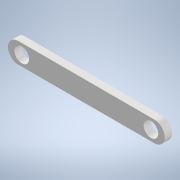
# Autodesk Inventor part: crank part
Saved by Autodesk Inventor 2022 (Build 260153070, 153G)
## iProperties
Created: 2021-07-24
Part Number: crank part
Material: Generic
Document SubType Name: Sheet Metal
Designer: DELL
Density: 1 g/cm^3
Sheet Metal Rule: Default
Appearance: Default
Author: DELL
Autodesk Inventor part; units mm, degrees
ref_plane "YZ Plane" through (0, 0, 0) normal (1, 0, 0) x (0, 1, 0)
ref_plane "XZ Plane" through (0, 0, 0) normal (0, 1, 0) x (-1, 0, 0)
ref_plane "XY Plane" through (0, 0, 0) normal (0, 0, 1) x (1, 0, 0)
sketch "Sketch1" plane through (0, 0, 0) normal (0, 0, 1) x (1, 0, 0)
  line L0 (-87.95, 8.89) -> (87.95, 8.89)
  line L1 (87.95, 8.89) -> (87.95, -8.89)
  line L2 (87.95, -8.89) -> (-87.95, -8.89)
  line L3 (-87.95, -8.89) -> (-87.95, 8.89)
  line L4 (-87.95, 8.89) -> (87.95, -8.89) construction
  line L5 (87.95, 8.89) -> (-87.95, -8.89) construction
  point P0 (0, 0)
  dimension "d0" = 175.9
  dimension "d1" = 17.78
  constraints: 12 end point, 2 midpoint, 2 parallel, 1 horizontal, 1 perpendicular
  measures "d0" distance of L1.end L2.end
  measures "d1" distance of L0.end L1.end
extrude "Extrusion1" add sketch "Sketch1" along normal blind 6.35
fillet "Fillet1" radius 8.89 1 edges at (87.95, 8.89, 3.175)
fillet "Fillet2" radius 8.89 1 edges at (87.95, -8.89, 3.175)
fillet "Fillet3" radius 8.89 1 edges at (-87.95, -8.89, 3.175)
fillet "Fillet4" radius 8.89 1 edges at (-87.95, 8.89, 3.175)
sketch "Sketch2" plane through (0, 0, 6.35) normal (0, 0, 1) x (1, 0, 0)
  arc A0 (79.06, -8.89) -> (79.06, 8.89) centre (79.06, 0) ccw projected
  circle A1 centre (-75.96, 0) radius 6.35
  circle A2 centre (75.96, 0) radius 6.35
  arc A3 (-79.06, 8.89) -> (-79.06, -8.89) centre (-79.06, 0) ccw projected
  point P0 (0, 0)
  dimension "d10" = 12.7
  dimension "d12" = 12.7
  dimension "d13" = 3.1
  dimension "d14" = 3.1
  constraints: 2 centre point
  measures "d10" diameter of A1
  measures "d12" diameter of A2
  measures "d13" distance of A0.centre A2.centre
  measures "d14" distance of A3.centre A1.centre
hole "Hole1" at (-75.96, 0, 6.35) at (75.96, 0, 6.35) direction (0, 0, -1) diameter 12.7 end through all
equation "\"d20\" = Thickness"
equation "\"BendRadius\" = Thickness"
equation "\"BendReliefWidth\" = Thickness"
equation "\"BendReliefDepth\" = 0.5 * Thickness"
equation "\"CornerReliefSize\" = 4 * Thickness"
equation "\"MinimumRemnant\" = 2 * Thickness"
equation "\"TransitionRadius\" = BendRadius"
equation "\"JacobiRadiusSize\" = BendRadius"
equation "\"GapSize\" = Thickness"
equation "\"Thickness\" = 3.048"
body "Solid1"
